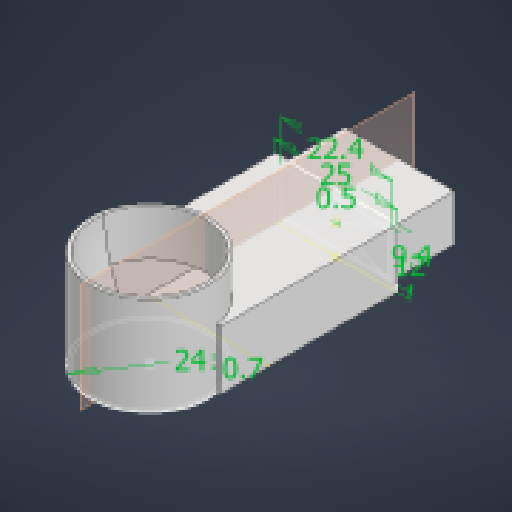
# Autodesk Inventor part: Wire_aisle_v1
Saved by Autodesk Inventor 2026.1 (Build 301233020, 233B)
## iProperties
Created: 2025-12-03
Part Number: Wire_aisle_v1
Material: 일반
Document SubType Name: Modeling
Designer: jaewook
Density: 1 g/cm^3
Appearance: 기본값
Author: jaewook
Autodesk Inventor part; units mm, degrees
ref_plane "YZ Plane" through (0, 0, 0) normal (1, 0, 0) x (0, 1, 0)
ref_plane "XZ Plane" through (0, 0, 0) normal (0, 1, 0) x (-1, 0, 0)
ref_plane "XY Plane" through (0, 0, 0) normal (0, 0, 1) x (1, 0, 0)
sketch "스케치1" plane through (0, 0, 0) normal (0, 0, 1) x (1, 0, 0)
  line L0 (-11.2, -4.7) -> (11.2, -4.7)
  line L1 (11.2, -4.7) -> (11.2, 4.7)
  line L2 (11.2, 4.7) -> (-11.2, 4.7)
  line L3 (-11.2, 4.7) -> (-11.2, -4.7)
  line L4 (-11.2, -4.7) -> (11.2, 4.7) construction
  line L5 (11.2, -4.7) -> (-11.2, 4.7) construction
  line L6 (-12.5, -6) -> (12.5, -6)
  line L7 (12.5, -6) -> (12.5, 6)
  line L8 (12.5, 6) -> (-12.5, 6)
  line L9 (-12.5, 6) -> (-12.5, -6)
  line L10 (-12.5, -6) -> (12.5, 6) construction
  line L11 (12.5, -6) -> (-12.5, 6) construction
  line L12 (-10.7, 4.2) -> (10.7, 4.2)
  line L13 (10.7, 4.2) -> (10.7, -4.2)
  line L14 (10.7, -4.2) -> (-10.7, -4.2)
  line L15 (-10.7, -4.2) -> (-10.7, 4.2)
  point P0 (0, 0)
  dimension "d0" = 22.4
  dimension "d1" = 9.4
  dimension "d2" = 25
  dimension "d3" = 12
  dimension "d6" = 0.5
  constraints: 32 end point, 6 parallel, 4 midpoint, 3 perpendicular, 2 horizontal, 3 other
  measures "d0" distance of L1.end L2.end
  measures "d1" distance of L0.end L1.end
  measures "d2" distance of L8.end L7.end
  measures "d3" distance of L7.end L6.end
  measures "d6" distance between parallel lines of L2 L12
extrude "돌출1" add sketch "스케치1" along normal blind 25.5 contours L9 L8 L7 L6
extrude "돌출2" add sketch "스케치1" against normal blind 13 contours L3 L2 L1 L0
sketch "스케치2" plane through (-12.5, -6, 0) normal (0, -1, 0) x (1, 0, 0)
  line L0 (0, 0) -> (25, 0) projected
  line L1 (0, 25.5) -> (25, 25.5) projected
  circle A0 centre (12.5, 37.5) radius 12
  circle A1 centre (12.5, 37.5) radius 11.3
  point P0 (12.5, 0)
  point P1 (12.5, 0)
  dimension "d9" = 24
  dimension "d11" = 0.7
  constraints: 2 centre point, 1 midpoint, 1 tangent, 1 vertical alignment
  measures "d9" diameter of A0
  measures "d11" radial gap between concentric circles of A0 A1
extrude "돌출3" add sketch "스케치2" against normal blind 20 contours A0 | A1
sketch "스케치3" plane through (0, 0, 25.5) normal (0, 0, 1) x (1, 0, 0)
  line L0 (0, -6) -> (12.5, -6) projected
  line L1 (12.5, -6) -> (12.5, 6) projected
  line L2 (12.5, 6) -> (0, 6) projected
  line L3 (0, 4.7) -> (11.2, 4.7) projected
  line L4 (11.2, 4.7) -> (11.2, -4.7) projected
  line L5 (11.2, -4.7) -> (0, -4.7) projected
  line L6 (0, -6) -> (0, -4.7) projected
  line L7 (0, -4.7) -> (-11.2, -4.7) projected
  line L8 (-11.2, -4.7) -> (-11.2, 4.7) projected
  line L9 (-11.2, 4.7) -> (0, 4.7) projected
  line L10 (0, 4.7) -> (0, 6) projected
  line L11 (0, 6) -> (-12.5, 6) projected
  line L12 (-12.5, 6) -> (-12.5, -6) projected
  line L13 (-12.5, -6) -> (0, -6) projected
  line L14 (0, -6) -> (12.5, -6) projected
  line L15 (12.5, -6) -> (12.5, 6) projected
  line L16 (12.5, 6) -> (0, 6) projected
  line L17 (0, 4.7) -> (11.2, 4.7) projected
  line L18 (11.2, 4.7) -> (11.2, -4.7) projected
  line L19 (11.2, -4.7) -> (0, -4.7) projected
  point P0 (0, 0)
extrude "돌출4" add sketch "스케치3" along normal blind 10 contours L6 L5 L4 L3 L10 L2 L1 L0 | L13 L12 L11 L10 L9 L8 L7 L6
extrude "돌출5" cut sketch "스케치2" along normal blind 19 from surface at -20 contours A1
extrude "돌출6" cut sketch "스케치1" along normal blind 35 contours L3 L2 L1 L0 | L12 L13 L14 L15
ref_plane "작업 평면1" through (0, -6, 0) normal (1, 0, 0) x (0, 0, -1)
sketch "스케치4" plane through (0, -6, 0) normal (1, 0, 0) x (0, 0, -1)
  line L0 (-26.2, 20) -> (-26.2, 1) projected
  line L1 (-26.2, 20) -> (-26.2, 1) projected
  line L2 (0, 10.7) -> (-35, 10.7) projected
  line L3 (-48.8, 20) -> (-48.8, 1) projected
  line L4 (-26.2, 1) -> (-48.8, 1) projected
  line L5 (-26.2, 20) -> (-26.2, 1.2542)
  line L6 (-48.8, 20) -> (-26.2, 20)
  line L7 (-37.5, 1) -> (-37.5, 20)
  arc A0 (-48.8, 20) -> (-38.437, 0.9996) centre (-26.2, 20) ccw
  point P0 (0, 6)
  point P1 (-38.4376, 1)
  constraints: 6 end point, 2 coincident, 2 midpoint, 2 point on circle, 1 centre point, 1 horizontal, 1 point on line, 1 vertical
revolve "회전1" add sketch "스케치4" angle 200 mid plane about axis through (0, -5, 37.5) along (0, 1, 0) contours L4 L3 A0
